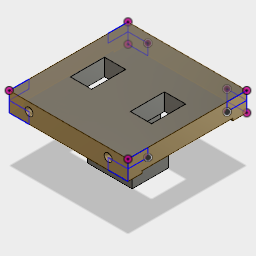
power_switch_holder (Autodesk Fusion 360 design; units mm, degrees)
Autodesk Fusion 360 part; units mm, degrees
sketch "スケッチ1" plane through (0, 0, 0) normal (0, 1, 0) x (1, 0, 0)
  line L0 (12.8775, 12.88) -> (-12.8775, 12.88)
  line L1 (-12.8775, 12.88) -> (-12.8775, -12.88)
  line L2 (-12.8775, -12.88) -> (12.8775, -12.88)
  line L3 (12.8775, -12.88) -> (12.8775, 12.88)
  line L4 (12.8775, 12.88) -> (-12.8775, -12.88) construction
  line L5 (-12.8775, 12.88) -> (12.8775, -12.88) construction
  line L6 (4.85, -3.95) -> (-4.85, -3.95)
  line L7 (-4.85, -3.95) -> (-4.85, 3.95)
  line L8 (-4.85, 3.95) -> (4.85, 3.95)
  line L9 (4.85, 3.95) -> (4.85, -3.95)
  line L10 (4.85, -3.95) -> (-4.85, 3.95) construction
  line L11 (-4.85, -3.95) -> (4.85, 3.95) construction
  line L12 (3.1275, -3.95) -> (-3.1275, -3.95)
  line L13 (-3.1275, -3.95) -> (-3.1275, 3.95)
  line L14 (-3.1275, 3.95) -> (3.1275, 3.95)
  line L15 (3.1275, 3.95) -> (3.1275, -3.95)
  line L16 (3.1275, -3.95) -> (-3.1275, 3.95) construction
  line L17 (-3.1275, -3.95) -> (3.1275, 3.95) construction
  line L18 (12.8775, 9.825) -> (-12.8775, 9.825)
  line L19 (-12.8775, 9.825) -> (-12.8775, -9.825)
  line L20 (-12.8775, -9.825) -> (12.8775, -9.825)
  line L21 (12.8775, -9.825) -> (12.8775, 9.825)
  line L22 (12.8775, 9.825) -> (-12.8775, -9.825) construction
  line L23 (-12.8775, 9.825) -> (12.8775, -9.825) construction
  dimension "d1" = 25.755
  dimension "d2" = 25.76
  dimension "d3" = 9.7
  dimension "d4" = 7.9
  dimension "d5" = 6.255
  dimension "d6" = 7.9
  dimension "d7" = 25.755
  dimension "d8" = 19.65
  constraint perpendicular L0 L1
  constraint parallel L0 L2
  constraint parallel L1 L3
  constraint horizontal L0
  constraint coincident L4
  constraint coincident L5
  constraint perpendicular L6 L7
  constraint parallel L6 L8
  constraint parallel L7 L9
  constraint horizontal L6
  constraint coincident L10
  constraint coincident L11
  constraint perpendicular L12 L13
  constraint parallel L12 L14
  constraint parallel L13 L15
  constraint horizontal L12
  constraint coincident L16
  constraint coincident L17
  constraint perpendicular L18 L19
  constraint parallel L18 L20
  constraint parallel L19 L21
  constraint horizontal L18
  constraint coincident L22
  constraint coincident L23
sketch "スケッチ2" plane through (0, 0, 0) normal (0, 1, 0) x (1, 0, 0)
  line L0 (0, 0) -> (-6.5, 0)
  line L1 (0, 0) -> (6.5, 0) construction
  line L2 (3.1275, 3.95) -> (3.1275, -3.95)
  line L3 (0, 0) -> (6.5, 0)
  line L4 (-4.2, -3.7) -> (-8.8, -3.7)
  line L5 (-8.8, -3.7) -> (-8.8, 3.7)
  line L6 (-8.8, 3.7) -> (-4.2, 3.7)
  line L7 (-4.2, 3.7) -> (-4.2, -3.7)
  line L8 (-4.2, -3.7) -> (-8.8, 3.7) construction
  line L9 (-8.8, -3.7) -> (-4.2, 3.7) construction
  line L10 (8.8, -3.7) -> (4.2, -3.7)
  line L11 (4.2, -3.7) -> (4.2, 3.7)
  line L12 (4.2, 3.7) -> (8.8, 3.7)
  line L13 (8.8, 3.7) -> (8.8, -3.7)
  line L14 (8.8, -3.7) -> (4.2, 3.7) construction
  line L15 (4.2, -3.7) -> (8.8, 3.7) construction
  dimension "d9" = 180
  dimension "d10" = 6.5
  dimension "d11" = 4.6
  dimension "d12" = 7.4
  dimension "d13" = 4.6
  dimension "d14" = 7.4
  constraint horizontal L1
  constraint perpendicular L2 L3
  constraint perpendicular L4 L5
  constraint parallel L4 L6
  constraint parallel L5 L7
  constraint horizontal L4
  constraint coincident L8
  constraint coincident L9
  constraint perpendicular L10 L11
  constraint parallel L10 L12
  constraint parallel L11 L13
  constraint horizontal L10
  constraint coincident L14
  constraint coincident L15
  measures "d9" angle of L0 L1
extrude "押し出し1" add sketch "スケッチ1" along normal blind 3.7 contours L0 L1 L3 L18 | L1 L3 L18 L19 L20 L21 | L1 L2 L3 L20 | L6 L8 L9 L15 | L6 L8 L12 L13 L14 L15 | L6 L7 L8 L13
extrude "押し出し2" add sketch "スケッチ1" against normal blind 0.5 contours L0 L1 L3 L18 | L1 L2 L3 L20
extrude "押し出し3" add sketch "スケッチ1" against normal blind 10.4 contours L6 L8 L9 L15 | L6 L8 L12 L13 L14 L15 | L6 L7 L8 L13
extrude "押し出し4" cut sketch "スケッチ1" against normal blind 7.4 contours L6 L8 L9 L15 | L6 L7 L8 L13
extrude "押し出し5" cut sketch "スケッチ2" along normal blind 4
sketch "スケッチ3" plane through (0, 0, 12.88) normal (0, 0, 1) x (1, 0, 0)
  line L0 (12.8775, -0.5) -> (12.8775, 3.7)
  line L1 (12.8775, 3.7) -> (-12.8775, 3.7)
  line L2 (-12.8775, 3.7) -> (-12.8775, -0.5)
  line L3 (-12.8775, -0.5) -> (12.8775, -0.5)
  line L4 (-12.8775, -0.5) -> (-8.5775, -0.5)
  line L5 (-8.5775, -0.5) -> (-8.5775, 1.85)
  line L6 (-8.5775, 1.85) -> (-12.8775, 1.85)
  line L7 (-12.8775, 1.85) -> (-12.8775, -0.5)
  line L8 (12.8775, -0.5) -> (8.5775, -0.5)
  line L9 (8.5775, -0.5) -> (8.5775, 1.85)
  line L10 (8.5775, 1.85) -> (12.8775, 1.85)
  line L11 (12.8775, 1.85) -> (12.8775, -0.5)
  dimension "d25" = 4.3
  dimension "d26" = 2.35
  dimension "d27" = 4.3
  dimension "d28" = 2.35
  constraint vertical L5
  constraint horizontal L6
  constraint horizontal L8
  constraint vertical L9
  constraint horizontal L10
  constraint vertical L11
sketch "スケッチ4" plane through (0, 0, -12.88) normal (0, 0, -1) x (-1, 0, 0)
  line L0 (12.8775, -0.5) -> (12.8775, 3.7)
  line L1 (12.8775, 3.7) -> (-12.8775, 3.7)
  line L2 (-12.8775, 3.7) -> (-12.8775, -0.5)
  line L3 (-12.8775, -0.5) -> (12.8775, -0.5)
  line L4 (12.8775, -0.5) -> (8.5775, -0.5)
  line L5 (8.5775, -0.5) -> (8.5775, 1.85)
  line L6 (8.5775, 1.85) -> (12.8775, 1.85)
  line L7 (12.8775, 1.85) -> (12.8775, -0.5)
  line L8 (-12.8775, -0.5) -> (-8.5775, -0.5)
  line L9 (-8.5775, -0.5) -> (-8.5775, 1.85)
  line L10 (-8.5775, 1.85) -> (-12.8775, 1.85)
  line L11 (-12.8775, 1.85) -> (-12.8775, -0.5)
  constraint horizontal L4
  constraint vertical L5
  constraint horizontal L6
  constraint vertical L7
  constraint horizontal L8
  constraint vertical L9
  constraint horizontal L10
  constraint vertical L11
sketch "スケッチ5" plane through (-12.8775, 0, 0) normal (-1, 0, 0) x (0, 0, 1)
  line L0 (-9.825, 0) -> (9.825, 0)
  line L1 (9.825, 0) -> (9.825, -0.5)
  line L2 (9.825, -0.5) -> (12.88, -0.5)
  line L3 (12.88, -0.5) -> (12.88, 3.7)
  line L4 (12.88, 3.7) -> (-12.88, 3.7)
  line L5 (-12.88, 3.7) -> (-12.88, -0.5)
  line L6 (-12.88, -0.5) -> (-9.825, -0.5)
  line L7 (-9.825, -0.5) -> (-9.825, 0)
  line L8 (12.88, 3.7) -> (8.58, 3.7)
  line L9 (8.58, 3.7) -> (8.58, 1.85)
  line L10 (8.58, 1.85) -> (12.88, 1.85)
  line L11 (12.88, 1.85) -> (12.88, 3.7)
  line L12 (-12.88, 3.7) -> (-8.58, 3.7)
  line L13 (-8.58, 3.7) -> (-8.58, 1.85)
  line L14 (-8.58, 1.85) -> (-12.88, 1.85)
  line L15 (-12.88, 1.85) -> (-12.88, 3.7)
  dimension "d29" = 4.3
  dimension "d30" = 1.85
  dimension "d31" = 4.3
  dimension "d32" = 1.85
  constraint horizontal L8
  constraint vertical L9
  constraint horizontal L10
  constraint vertical L11
  constraint horizontal L12
  constraint vertical L13
  constraint horizontal L14
  constraint vertical L15
sketch "スケッチ6" plane through (12.8775, 0, 0) normal (1, 0, 0) x (0, 0, -1)
  line L0 (-9.825, 0) -> (9.825, 0)
  line L1 (9.825, 0) -> (9.825, -0.5)
  line L2 (9.825, -0.5) -> (12.88, -0.5)
  line L3 (12.88, -0.5) -> (12.88, 3.7)
  line L4 (12.88, 3.7) -> (-12.88, 3.7)
  line L5 (-12.88, 3.7) -> (-12.88, -0.5)
  line L6 (-12.88, -0.5) -> (-9.825, -0.5)
  line L7 (-9.825, -0.5) -> (-9.825, 0)
  line L8 (12.88, 3.7) -> (8.58, 3.7)
  line L9 (8.58, 3.7) -> (8.58, 1.85)
  line L10 (8.58, 1.85) -> (12.88, 1.85)
  line L11 (12.88, 1.85) -> (12.88, 3.7)
  line L12 (-12.88, 3.7) -> (-8.58, 3.7)
  line L13 (-8.58, 3.7) -> (-8.58, 1.85)
  line L14 (-8.58, 1.85) -> (-12.88, 1.85)
  line L15 (-12.88, 1.85) -> (-12.88, 3.7)
  constraint horizontal L8
  constraint vertical L9
  constraint horizontal L10
  constraint vertical L11
  constraint horizontal L12
  constraint vertical L13
  constraint horizontal L14
  constraint vertical L15
sphere "球プリミティブ1" cut diameter 1.7 placed x (1, 0, 0) y (0, 1, 0) z (0, 0, 1) at (-8.5775, 1.85, 12.88)
sphere "球プリミティブ2" cut diameter 1.7 placed x (1, 0, 0) y (0, 1, 0) z (0, 0, 1) at (8.5775, 1.85, 12.88)
sphere "球プリミティブ3" cut diameter 1.7 placed x (-1, 0, 0) y (0, 1, 0) z (0, 0, -1) at (-8.5775, 1.85, -12.88)
sphere "球プリミティブ4" cut diameter 1.7 placed x (-1, 0, 0) y (0, 1, 0) z (0, 0, -1) at (8.5775, 1.85, -12.88)
sphereprimitive "球プリミティブ5" [suppressed]
sphereprimitive "球プリミティブ6" [suppressed]
sphereprimitive "球プリミティブ7" [suppressed]
sphereprimitive "球プリミティブ8" [suppressed]
